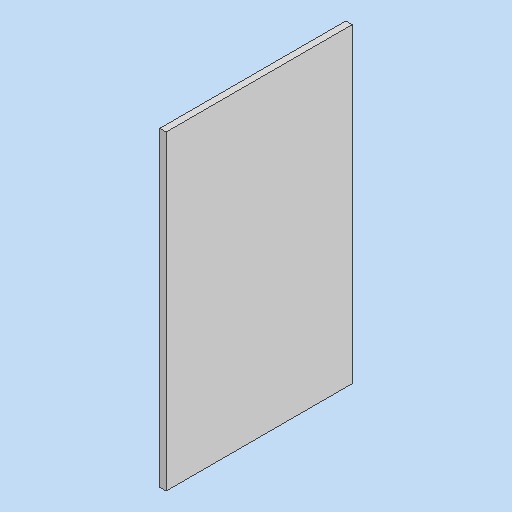
# Autodesk Inventor part: inside walls front
Saved by Autodesk Inventor 2026 (Build 300175000, 175)
## iProperties
Created: 2026-02-03
Part Number: inside walls front
Material: Generic
Document SubType Name: Modeling
Designer: mones
Density: 1 g/cm^3
Appearance: Default
Author: mones
Autodesk Inventor part; units mm, degrees
ref_plane "YZ Plane" through (0, 0, 0) normal (1, 0, 0) x (0, 1, 0)
ref_plane "XZ Plane" through (0, 0, 0) normal (0, 1, 0) x (-1, 0, 0)
ref_plane "XY Plane" through (0, 0, 0) normal (0, 0, 1) x (1, 0, 0)
sketch "Sketch1" plane through (0, 0, 0) normal (1, 0, 0) x (0, 1, 0)
  line L0 (98.5, 44) -> (98.5, -44)
  line L1 (98.5, -44) -> (-48.5, -44)
  line L2 (-48.5, -44) -> (-48.5, 44)
  line L3 (-48.5, 44) -> (98.5, 44)
  line L4 (98.5, 44) -> (-48.5, -44) construction
  line L5 (98.5, -44) -> (-48.5, 44) construction
  point P0 (25, 0)
  dimension "d0" = 88
  dimension "d1" = 147
  constraints: 12 end point, 2 midpoint, 2 parallel, 1 perpendicular, 1 vertical
  measures "d0" distance of L0.start L0.end
  measures "d1" distance of L0.end L1.end
extrude "Extrusion1" add sketch "Sketch1" along normal blind 3
body "Solid1"
